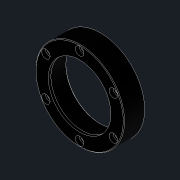
# Autodesk Inventor part: bearing_cover_j5
Saved by Autodesk Inventor 2022 (Build 260153000, 153)
## iProperties
Created: 2021-07-25
Part Number: bearing_cover_j5
Material: ABS プラスチック
Document SubType Name: Modeling
Designer: yuto6
Density: 1.06 g/cm^3
Appearance: 滑らか - 黒
Mass: 24.8073 g
Surface Area: 106.323 cm^2
Volume: 23.4032 cm^3
購入先: 印刷
在庫数: 0.0
Author: yuto6
Autodesk Inventor part; units mm, degrees
ref_plane "YZ Plane" through (0, 0, 0) normal (1, 0, 0) x (0, 1, 0)
ref_plane "XZ Plane" through (0, 0, 0) normal (0, 1, 0) x (-1, 0, 0)
ref_plane "XY Plane" through (0, 0, 0) normal (0, 0, 1) x (1, 0, 0)
sketch "スケッチ2" plane through (0, 0, 0) normal (1, 0, 0) x (0, 1, 0)
  line L0 (0, 0) -> (26.1, 0)
  line L1 (26.1, 0) -> (26.1, -16)
  line L2 (26.1, -16) -> (0, -16)
  line L3 (0, -16) -> (0, 0)
  line L4 (0, 0) -> (34.1, 0)
  line L5 (34.1, 0) -> (34.1, -16)
  line L6 (34.1, -16) -> (0, -16)
  line L7 (0, -16) -> (0, 0)
  line L8 (34.1, 0) -> (21, 0)
  line L9 (26.1, 0) -> (24.1, 0)
  line L10 (24.1, 0) -> (24.1, -2)
  line L11 (24.1, -2) -> (26.1, -2)
  line L12 (26.1, -2) -> (26.1, 0)
  point P0 (26.1, 0)
  point P1 (24.1, 0)
  dimension "d1" = 26.1
  dimension "d8" = 2
  dimension "d10" = 14
  dimension "d27" = 8
  dimension "d31" = 2
  constraints: 26 end point, 6 parallel, 4 horizontal, 3 perpendicular, 1 point on line
  measures "d1" distance of L1.end L2.end
  measures "d8" distance of L9.end L10.end
  measures "d10" distance between parallel lines of L2 L11
  measures "d27" distance between parallel lines of L1 L5
  measures "d31" distance of L10.end L11.end
revolve "回転1" add sketch "スケッチ2" angle 360 about axis through (0, 0, -16) along (0, 0, 1) contours L0 L1 L11 L10 | L1 L4 L5 L6
sketch "スケッチ4" plane through (0, 0, 0) normal (0, 0, 1) x (1, 0, 0)
  point P0 (0, 0)
  point P1 (0, 30)
  point P2 (-25.9808, 15)
  point P3 (-25.9808, -15)
  point P4 (0, -30)
  point P5 (25.9808, -15)
  point P6 (25.9808, 15)
  dimension "d11" = 30
  dimension "d14" = 360
  constraints: 7 other
  measures "d11" distance of point (0, 0) point (0, 30)
hole "穴1" at (0, 30, 0) at (-25.9808, 15, 0) at (-25.9808, -15, 0) at (0, -30, 0) at (25.9808, -15, 0) at (25.9808, 15, 0) direction (0, 0, -1) diameter 3.4 end through all counterbore diameter 6.5 counterbore depth 3 clearance for "Socket Head Cap Screw" size "M3" standard "Ansi Metric M Profile"
chamfer "面取り1" distance 0.5 angle 45 1 edges at (0, -26.1, -16)
chamfer "面取り2" distance 0.5 angle 45 1 edges at (0, -34.1, 0)
